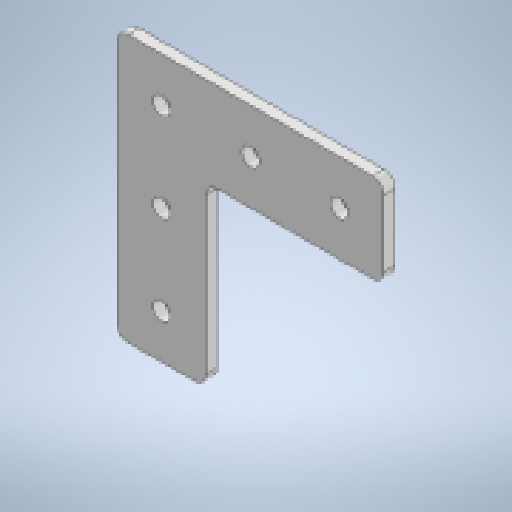
# Autodesk Inventor part: L_gusset
Saved by Autodesk Inventor 2024 (Build 280153000, 153)
## iProperties
Created: 2023-04-21
Part Number: L_gusset
Material: Aluminum 6061
Document SubType Name: Modeling
Designer: legom
Density: 2.7 g/cm^3
Appearance: Aluminum - Flat
Author: legom
Autodesk Inventor part; units mm, degrees
ref_plane "YZ Plane" through (0, 0, 0) normal (1, 0, 0) x (0, 1, 0)
ref_plane "XZ Plane" through (0, 0, 0) normal (0, 1, 0) x (-1, 0, 0)
ref_plane "XY Plane" through (0, 0, 0) normal (0, 0, 1) x (1, 0, 0)
sketch "Sketch1" plane through (0, 0, 0) normal (0, 0, 1) x (1, 0, 0)
  line L0 (0, 0) -> (76.2, 0)
  line L1 (76.2, 0) -> (76.2, -25.4)
  line L2 (76.2, -25.4) -> (0, -25.4)
  line L3 (0, -25.4) -> (0, 0)
  line L4 (0, -25.4) -> (25.4, -25.4)
  line L5 (25.4, -25.4) -> (25.4, -76.2)
  line L6 (25.4, -76.2) -> (0, -76.2)
  line L7 (0, -76.2) -> (0, -25.4)
  circle A0 centre (12.7, -12.7) radius 2.5527
  circle A1 centre (38.1, -12.7) radius 2.5527
  circle A2 centre (63.5, -12.7) radius 2.5527
  circle A3 centre (12.7, -38.1) radius 2.5527
  circle A4 centre (12.7, -63.5) radius 2.5527
  point P0 (0, -12.7)
  dimension "d0" = 76.2
  dimension "d1" = 25.4
  dimension "d2" = 25.4
  dimension "d3" = 50.8
  dimension "d4" = 5.1054
  dimension "d5" = 12.7
  dimension "d6" = 12.7
  dimension "d9" = 25.4
  dimension "d16" = 25.4
  constraints: 16 end point, 5 centre point, 4 parallel, 3 horizontal, 2 perpendicular, 1 midpoint, 1 vertical, 8 other
  measures "d0" distance of L1.end L2.end
  measures "d1" distance of L0.end L1.end
  measures "d2" distance of L5.end L6.end
  measures "d3" distance of L4.end L5.end
  measures "d4" diameter of A0
  measures "d5" distance from line of L0 A0.centre
  measures "d6" distance of point (0, -12.7) A0.centre
  measures "d9" distance of A0.centre A1.centre
  measures "d16" distance of A0.centre A3.centre
extrude "Extrusion1" add sketch "Sketch1" along normal blind 3.175
fillet "Fillet1" radius 3.175 6 edges at (25.4, -25.4, 1.5875) (0, 0, 1.5875) (25.4, -76.2, 1.5875) (0, -76.2, 1.5875) (76.2, -25.4, 1.5875) (76.2, 0, 1.5875)
body "Solid1"
